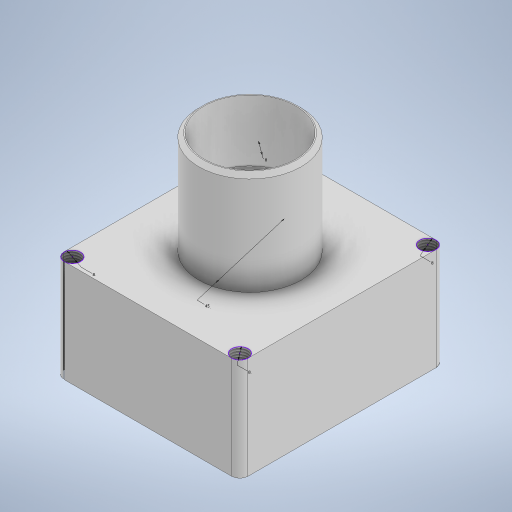
# Autodesk Inventor part: P#1_LAB_DINAMICA
Saved by Autodesk Inventor 2024 (Build 280153000, 153)
## iProperties
Created: 2024-01-22
Part Number: P#1_LAB_DINAMICA
Material: Generic
Document SubType Name: Modeling
Designer: HP15BW010LA
Density: 1 g/cm^3
Appearance: Default
Author: HP15BW010LA
Autodesk Inventor part; units mm, degrees
ref_plane "YZ Plane" through (0, 0, 0) normal (1, 0, 0) x (0, 1, 0)
ref_plane "XZ Plane" through (0, 0, 0) normal (0, 1, 0) x (-1, 0, 0)
ref_plane "XY Plane" through (0, 0, 0) normal (0, 0, 1) x (1, 0, 0)
sketch "Sketch1" plane through (0, 0, 0) normal (0, 1, 0) x (-1, 0, 0)
  line L0 (45, 50) -> (-45, 50)
  line L1 (-45, 50) -> (-45, -50)
  line L2 (-45, -50) -> (45, -50)
  line L3 (45, -50) -> (45, 50)
  line L4 (45, 50) -> (-45, -50) construction
  line L5 (-45, 50) -> (45, -50) construction
  point P0 (0, 0)
  point P1 (42.3062, 47.0069)
  point P2 (42.3062, -47.0069)
  point P3 (-42.3062, -47.0069)
  point P4 (-42.3062, 47.0069)
  dimension "d0" = 90
  dimension "d1" = 100
  constraints: 12 end point, 4 point on line, 2 midpoint, 2 parallel, 1 horizontal, 1 perpendicular
  measures "d0" distance of L2.end L1.end
  measures "d1" distance of L1.end L0.end
extrude "Extrusion1" add sketch "Sketch1" along normal blind 50
sketch "Sketch2" plane through (0, 50, 0) normal (0, 1, 0) x (1, 0, 0)
  circle A0 centre (0, 0) radius 25
  dimension "d5" = 50
  constraints: 1 centre point, 1 coincident
  measures "d5" diameter of A0
extrude "Extrusion2" add sketch "Sketch2" along normal blind 50
sketch "Sketch3" plane through (0, 50, 0) normal (0, 1, 0) x (1, 0, 0)
  point P0 (0, 0)
fillet "Fillet1" radius 4 1 edges at (45, 25, 50)
fillet "Fillet2" radius 4 3 edges at (-45, 25, 50) (45, 25, -50) (-45, 25, -50)
sketch "Sketch4" plane through (0, 50, 0) normal (0, 1, 0) x (1, 0, 0)
  circle A0 centre (-40.9319, 45.9787) radius 4
  circle A1 centre (40.8995, 45.9787) radius 4
  circle A2 centre (40.8995, -45.9186) radius 4
  circle A3 centre (-40.9319, -46.0049) radius 4
  point P0 (0, 0)
  dimension "d20" = 8
  dimension "d21" = 8
  dimension "d22" = 8
  dimension "d23" = 8
  constraints: 4 centre point
  measures "d20" diameter of A0
  measures "d21" diameter of A1
  measures "d22" diameter of A2
  measures "d23" diameter of A3
sketch "Sketch5" plane through (0, 50, 0) normal (0, 1, 0) x (1, 0, 0)
  circle A0 centre (0, 0) radius 22.5
  dimension "d16" = 45
  constraints: 1 centre point, 1 coincident
  measures "d16" diameter of A0
sketch "Sketch6" plane through (0, 100, 0) normal (0, 1, 0) x (1, 0, 0)
  circle A0 centre (0, 0) radius 22.5
  dimension "d17" = 45
  constraints: 1 centre point, 1 coincident
  measures "d17" diameter of A0
extrude "Extrusion3" cut sketch "Sketch6" against normal blind 30
sketch "Sketch7" plane through (0, 50, 0) normal (0, 1, 0) x (1, 0, 0)
  point P0 (0, 0)
sketch "Sketch8" plane through (0, 50, 0) normal (0, 1, 0) x (1, 0, 0)
  point P0 (0, 0)
hole "Hole1" at (40.8995, 50, 45.9186) direction (0, -1, 0) diameter 8 end through all
hole "Hole2" at (40.8995, 50, -45.9787) direction (0, -1, 0) diameter 8 end through all
hole "Hole3" at (-40.9319, 50, 46.0049) direction (0, -1, 0) diameter 8 end through all
hole "Hole4" at (-40.9319, 50, -45.9787) direction (0, -1, 0) diameter 8 end through all
thread "Thread1" size "M8x1.25" class "6H" standard "ANSI Metric M Profile" full length
thread "Thread2" size "M8x1.25" class "6H" standard "ANSI Metric M Profile" full length
thread "Thread3" size "M8x1.25" class "6H" standard "ANSI Metric M Profile" full length
thread "Thread4" size "M8x1.25" class "6H" standard "ANSI Metric M Profile" full length
chamfer "Chamfer1" distance 2 angle 45 1 edges at (-25, 100, 0)
sketch "Sketch9" plane through (0, 50, 0) normal (0, 1, 0) x (1, 0, 0)
  point P0 (0, 0)
body "Solid1"
